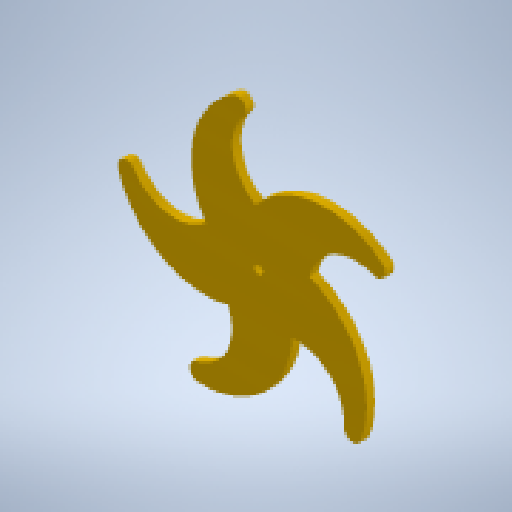
# Autodesk Inventor part: fan
Saved by Autodesk Inventor 2023 (Build 270158000, 158)
## iProperties
Created: 2023-03-24
Part Number: fan
Material: Generic
Document SubType Name: Modeling
Designer: AggyT
Density: 1 g/cm^3
Appearance: Gold
Author: AggyT
Autodesk Inventor part; units mm, degrees
ref_plane "YZ Plane" through (0, 0, 0) normal (1, 0, 0) x (0, 1, 0)
ref_plane "XZ Plane" through (0, 0, 0) normal (0, 1, 0) x (-1, 0, 0)
ref_plane "Work Plane2" through (0, 0, 25.4) normal (0, 0, 1) x (1, 0, 0)
sketch "Sketch2" plane through (0, 0, 25.4) normal (0, 0, 1) x (1, 0, 0)
  arc A0 (46.0596, 25.0506) -> (-2.2984, 18.6014) centre (24.9372, -1.0935) ccw
  arc A1 (42.8607, 19.6429) -> (18.6627, 1.7307) centre (36.1883, 3.3559) ccw
  arc A2 (42.8607, 19.6429) -> (46.0596, 25.0506) centre (44.0643, 22.5809) ccw
  circle A3 centre (0, 0) radius 18.7428
  arc A4 (-9.5913, 51.5464) -> (-18.4012, 3.5622) centre (8.746, 23.3788) ccw
  arc A5 (-5.4368, 46.8329) -> (-9.5913, 51.5464) centre (-7.8591, 48.8855) ccw
  arc A6 (-5.4368, 46.8329) -> (4.1211, 18.2841) centre (7.9911, 35.4541) ccw
  circle A7 centre (0, 0) radius 18.7428
  arc A8 (-51.9874, 6.8069) -> (-9.0742, -16.3998) centre (-19.5319, 15.5424) ccw
  arc A9 (-46.2208, 9.3015) -> (-51.9874, 6.8069) centre (-48.9215, 7.6321) ccw
  arc A10 (-46.2208, 9.3015) -> (-16.1158, 9.5695) centre (-31.2495, 18.5559) ccw
  circle A11 centre (0, 0) radius 18.7428
  arc A12 (-22.5387, -47.3395) -> (12.7931, -13.6979) centre (-20.8174, -13.7731) ccw
  arc A13 (-23.1292, -41.0843) -> (-22.5387, -47.3395) centre (-22.3761, -44.1687) ccw
  arc A14 (-23.1292, -41.0843) -> (-14.0812, -12.3698) centre (-27.3044, -23.9859) ccw
  circle A15 centre (0, 0) radius 18.7428
  arc A16 (38.0577, -36.0643) -> (16.9807, 7.9341) centre (6.666, -24.0546) ccw
  arc A17 (31.9262, -34.693) -> (38.0577, -36.0643) centre (35.0923, -34.9298) ccw
  arc A18 (31.9262, -34.693) -> (7.4131, -17.2145) centre (14.3745, -33.3801) ccw
  circle A19 centre (0, 0) radius 18.7428
  point P0 (18.6202, 2.2848)
  point P1 (-0.9774, 20.3098)
  point P2 (-19.6178, 5.3465)
  point P3 (-11.1471, -17.0054)
  point P4 (-18.4012, 3.5622)
  point P5 (-9.0742, -16.3998)
  point P6 (-14.0812, -12.3698)
  point P7 (12.7931, -13.6979)
  point P8 (12.7285, -15.8565)
  point P9 (19.0137, 7.2056)
  dimension "d3" = 3.175
  dimension "d6" = 360
  constraints: 40 point on circle, 20 centre point, 3 tangent, 1 coincident, 61 other
  measures "d3" radius of A2
extrude "Extrusion3" add sketch "Sketch2" along normal blind 3.175
sketch "Sketch3" plane through (0, 0, 25.4) normal (0, 0, -1) x (-1, 0, 0)
  circle A0 centre (0, 0) radius 1.5635
  dimension "d12" = 3.127
  constraints: 1 centre point, 1 coincident
  measures "d12" diameter of A0
extrude "Extrusion4" cut sketch "Sketch3" against normal through all
body "Solid1"
